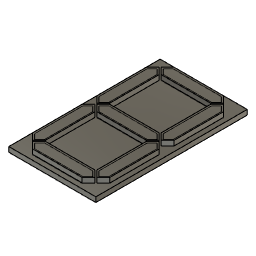
Digit (Autodesk Fusion 360 design; units mm, degrees)
Autodesk Fusion 360 part; units mm, degrees
note: some values were not read from the file. Set by a fixed rule: which face or edge a step refers to.
sketch "Esquisse1" plane through (0, 0, 0) normal (0, 0, 1) x (1, 0, 0)
  line L0 (25, 6.5) -> (-25, 6.5)
  line L1 (-25, 6.5) -> (-25, -6.5)
  line L2 (-25, -6.5) -> (25, -6.5)
  line L3 (25, -6.5) -> (25, 6.5)
  line L4 (25, 6.5) -> (-25, -6.5) construction
  line L5 (-25, 6.5) -> (25, -6.5) construction
  line L6 (-25, 6.5) -> (-25, -6.5) construction
  line L7 (-25, -6.5) -> (-31.5, -6.5) construction
  line L8 (-31.5, -6.5) -> (-31.5, 6.5) construction
  line L9 (-31.5, 6.5) -> (-25, 6.5) construction
  line L10 (-25, 6.5) -> (-31.5, 0)
  line L11 (-25, -6.5) -> (-31.5, 0)
  line L12 (25, 6.5) -> (25, -6.5) construction
  line L13 (25, -6.5) -> (31.5, -6.5) construction
  line L14 (31.5, -6.5) -> (31.5, 6.5) construction
  line L15 (31.5, 6.5) -> (25, 6.5) construction
  line L16 (25, 6.5) -> (31.5, 0)
  line L17 (25, -6.5) -> (31.5, 0)
  line L18 (-25, -6.5) -> (-25, -6.25) construction
  line L19 (-25, -6.25) -> (25, -6.25) construction
  line L20 (25, -6.25) -> (25, -6.5)
  line L21 (25, -6.5) -> (-25, -6.5)
  line L22 (-24.25, -6.25) -> (24.25, -6.25)
  line L23 (24.25, -6.25) -> (24.25, -5)
  line L24 (24.25, -5) -> (-24.25, -5)
  line L25 (-24.25, -5) -> (-24.25, -6.25)
  point P0 (-31.5, 0)
  point P1 (31.5, 0)
  dimension "longueurBande" = 50
  dimension "largeurBande" = 13
  dimension "d3" = 6.5
  dimension "d4" = 6.5
  dimension "d42" = 0.25
  dimension "d50" = 0.75
  dimension "d51" = 48.5
  dimension "d52" = 1.25
  constraint horizontal L0
  constraint perpendicular L0 L1
  constraint parallel L0 L2
  constraint parallel L1 L3
  constraint coincident L4 origin
  constraint coincident L5 origin
  constraint perpendicular L6 L7
  constraint parallel L6 L8
  constraint parallel L7 L9
  constraint midpoint L8 P0
  constraint coincident P0 L10.end
  constraint perpendicular L12 L13
  constraint parallel L12 L14
  constraint parallel L13 L15
  constraint midpoint L14 P1
  constraint coincident P1 L16.end
  constraint perpendicular L18 L19
  constraint parallel L18 L20
  constraint parallel L19 L21
  constraint coincident L1 L18.end
  constraint horizontal L22
  constraint vertical L23
  constraint horizontal L24
  constraint vertical L25
  constraint coincident L19 L22.start
  measures "longueurBande" distance of L1.end L2.end
  measures "largeurBande" distance of L0.end L1.end
  measures "d3" distance of L0.end L8.end
  measures "d4" distance of L0.start L14.end
  measures "d42" distance of L19 L21
  measures "d50" distance of L18.end L22.start
  measures "d51" distance of L23.end L24.end
  measures "d52" distance of L19 L24
extrude "Extrusion1" add sketch "Esquisse1" along normal blind 5 contours L0 L1 L2 L3 L20 L21 | L3 L16 L17 L20 | L1 L10 L11 | L22 L23 L24 L25 makes body 1
shell "Coque2" thickness 1.5 removed faces 1 at (8.3333, 2.1667, 0) on bodies 1
extrude "Extrusion10" cut 1 faces at (-8.1262, -1.6667, 3.5) along direction (0, 0, 1) blind 1 on bodies 1 bodies 1
extrude "Extrusion8" add sketch "Esquisse1" against normal blind 1 contours L22 L23 L24 L25 bodies 1
copy_body "Copier/Coller des corps2" bodies 1 makes body 2
move_body "Déplacer1" bodies 2 to x (0, -1, 0) y (1, 0, 0) z (0, 0, 1) at (-32.5, -32.5, 0)
pattern_linear "Réseau R1" count 3 spacing 65 along (0, -1, 0) of bodies 1 makes body 3 at (-8.3333, -67.1667, 5) makes body 4 at (-8.3333, -132.1667, 5)
pattern_linear "Réseau R2" count 2 spacing 65 along (1, 0, 0) count 2 spacing 65 along (0, -1, 0) of bodies 2 makes body 5 at (34.6667, -40.8333, 5) makes body 6 at (-30.3333, -105.8333, 5) makes body 7 at (34.6667, -105.8333, 5)
sketch "Esquisse2" plane through (0, 0, 0) normal (0, 0, 1) x (1, 0, 0)
  line L0 (-25, -6.5) -> (25, -6.5)
  line L1 (25, -6.5) -> (31.5, 0)
  line L2 (31.5, 0) -> (25, 6.5)
  line L3 (25, 6.5) -> (-25, 6.5)
  line L4 (-25, 6.5) -> (-31.5, 0)
  line L5 (-31.5, 0) -> (-25, -6.5)
  line L6 (26, -7.5) -> (26, -57.5)
  line L7 (26, -57.5) -> (32.5, -64)
  line L8 (32.5, -64) -> (39, -57.5)
  line L9 (39, -57.5) -> (39, -7.5)
  line L10 (39, -7.5) -> (32.5, -1)
  line L11 (32.5, -1) -> (26, -7.5)
  line L12 (-39, -7.5) -> (-39, -57.5)
  line L13 (-39, -57.5) -> (-32.5, -64)
  line L14 (-32.5, -64) -> (-26, -57.5)
  line L15 (-26, -57.5) -> (-26, -7.5)
  line L16 (-26, -7.5) -> (-32.5, -1)
  line L17 (-32.5, -1) -> (-39, -7.5)
  line L18 (-25, -71.5) -> (25, -71.5)
  line L19 (25, -71.5) -> (31.5, -65)
  line L20 (31.5, -65) -> (25, -58.5)
  line L21 (25, -58.5) -> (-25, -58.5)
  line L22 (-25, -58.5) -> (-31.5, -65)
  line L23 (-31.5, -65) -> (-25, -71.5)
  line L24 (-39, -72.5) -> (-39, -122.5)
  line L25 (-39, -122.5) -> (-32.5, -129)
  line L26 (-32.5, -129) -> (-26, -122.5)
  line L27 (-26, -122.5) -> (-26, -72.5)
  line L28 (-26, -72.5) -> (-32.5, -66)
  line L29 (-32.5, -66) -> (-39, -72.5)
  line L30 (26, -72.5) -> (26, -122.5)
  line L31 (26, -122.5) -> (32.5, -129)
  line L32 (32.5, -129) -> (39, -122.5)
  line L33 (39, -122.5) -> (39, -72.5)
  line L34 (39, -72.5) -> (32.5, -66)
  line L35 (32.5, -66) -> (26, -72.5)
  line L36 (-25, -136.5) -> (25, -136.5)
  line L37 (25, -136.5) -> (31.5, -130)
  line L38 (31.5, -130) -> (25, -123.5)
  line L39 (25, -123.5) -> (-25, -123.5)
  line L40 (-25, -123.5) -> (-31.5, -130)
  line L41 (-31.5, -130) -> (-25, -136.5)
  line L42 (-39, 6.5) -> (39, 6.5)
  line L43 (39, 6.5) -> (39, -136.5)
  line L44 (39, -136.5) -> (-39, -136.5)
  line L45 (-39, -136.5) -> (-39, 6.5)
  line L46 (44, 11.5) -> (44, -141.5)
  line L47 (44, -141.5) -> (-44, -141.5)
  line L48 (-44, -141.5) -> (-44, 11.5)
  line L49 (-44, 11.5) -> (44, 11.5)
  line L50 (-25, -6.5) -> (-26, -7.5)
  line L51 (31.5, 0) -> (32.5, -1)
  line L52 (25, -6.5) -> (26, -7.5)
  line L53 (26, -57.5) -> (25, -58.5)
  line L54 (32.5, -64) -> (31.5, -65)
  line L55 (31.5, -65) -> (32.5, -66)
  line L56 (25, -71.5) -> (26, -72.5)
  line L57 (26, -122.5) -> (25, -123.5)
  line L58 (32.5, -129) -> (31.5, -130)
  line L59 (-25, -123.5) -> (-26, -122.5)
  line L60 (-32.5, -129) -> (-31.5, -130)
  line L61 (-32.5, -66) -> (-31.5, -65)
  line L62 (-26, -72.5) -> (-25, -71.5)
  line L63 (-31.5, -65) -> (-32.5, -64)
  line L64 (-25, -58.5) -> (-26, -57.5)
  line L65 (-24.3787, -5) -> (24.3787, -5)
  line L66 (24.3787, -5) -> (29.3787, 0)
  line L67 (29.3787, 0) -> (24.3787, 5)
  line L68 (24.3787, 5) -> (-24.3787, 5)
  line L69 (-24.3787, 5) -> (-29.3787, 0)
  line L70 (-29.3787, 0) -> (-24.3787, -5)
  line L71 (-37.5, -56.8787) -> (-32.5, -61.8787)
  line L72 (-32.5, -61.8787) -> (-27.5, -56.8787)
  line L73 (-27.5, -56.8787) -> (-27.5, -8.1213)
  line L74 (-27.5, -8.1213) -> (-32.5, -3.1213)
  line L75 (-32.5, -3.1213) -> (-37.5, -8.1213)
  line L76 (-37.5, -8.1213) -> (-37.5, -56.8787)
  line L77 (27.5, -56.8787) -> (32.5, -61.8787)
  line L78 (32.5, -61.8787) -> (37.5, -56.8787)
  line L79 (37.5, -56.8787) -> (37.5, -8.1213)
  line L80 (37.5, -8.1213) -> (32.5, -3.1213)
  line L81 (32.5, -3.1213) -> (27.5, -8.1213)
  line L82 (27.5, -8.1213) -> (27.5, -56.8787)
  line L83 (-24.3787, -70) -> (24.3787, -70)
  line L84 (24.3787, -70) -> (29.3787, -65)
  line L85 (29.3787, -65) -> (24.3787, -60)
  line L86 (24.3787, -60) -> (-24.3787, -60)
  line L87 (-24.3787, -60) -> (-29.3787, -65)
  line L88 (-29.3787, -65) -> (-24.3787, -70)
  line L89 (27.5, -121.8787) -> (32.5, -126.8787)
  line L90 (32.5, -126.8787) -> (37.5, -121.8787)
  line L91 (37.5, -121.8787) -> (37.5, -73.1213)
  line L92 (37.5, -73.1213) -> (32.5, -68.1213)
  line L93 (32.5, -68.1213) -> (27.5, -73.1213)
  line L94 (27.5, -73.1213) -> (27.5, -121.8787)
  line L95 (-37.5, -121.8787) -> (-32.5, -126.8787)
  line L96 (-32.5, -126.8787) -> (-27.5, -121.8787)
  line L97 (-27.5, -121.8787) -> (-27.5, -73.1213)
  line L98 (-27.5, -73.1213) -> (-32.5, -68.1213)
  line L99 (-32.5, -68.1213) -> (-37.5, -73.1213)
  line L100 (-37.5, -73.1213) -> (-37.5, -121.8787)
  line L101 (-24.3787, -135) -> (24.3787, -135)
  line L102 (24.3787, -135) -> (29.3787, -130)
  line L103 (29.3787, -130) -> (24.3787, -125)
  line L104 (24.3787, -125) -> (-24.3787, -125)
  line L105 (-24.3787, -125) -> (-29.3787, -130)
  line L106 (-29.3787, -130) -> (-24.3787, -135)
  line L107 (-32.5, -3.1213) -> (-29.3787, 0)
  line L108 (-24.3787, -5) -> (-27.5, -8.1213)
  line L109 (24.3787, -5) -> (27.5, -8.1213)
  line L110 (32.5, -3.1213) -> (29.3787, 0)
  line L111 (27.5, -56.8787) -> (24.3787, -60)
  line L112 (32.5, -61.8787) -> (32.5, -68.1213)
  line L113 (27.5, -73.1213) -> (24.3787, -70)
  line L114 (27.5, -121.8787) -> (24.3787, -125)
  line L115 (32.5, -126.8787) -> (29.3787, -130)
  line L116 (-27.5, -121.8787) -> (-24.3787, -125)
  line L117 (-29.3787, -130) -> (-32.5, -126.8787)
  line L118 (-32.5, -61.8787) -> (-32.5, -68.1213)
  line L119 (-27.5, -73.1213) -> (-24.3787, -70)
  line L120 (-24.3787, -60) -> (-27.5, -56.8787)
  line L121 (-32.5, -68.1213) -> (-32.5, -61.8787)
  line L122 (-32.5, -61.8787) -> (-39, -61.8787)
  line L123 (-39, -61.8787) -> (-39, -68.1213)
  line L124 (-39, -68.1213) -> (-32.5, -68.1213)
  line L125 (32.5, -68.1213) -> (32.5, -61.8787)
  line L126 (32.5, -61.8787) -> (39, -61.8787)
  line L127 (39, -61.8787) -> (39, -68.1213)
  line L128 (39, -68.1213) -> (32.5, -68.1213)
  line L129 (-24.3787, 5) -> (24.3787, 5)
  line L130 (24.3787, 5) -> (24.3787, 6.5)
  line L131 (24.3787, 6.5) -> (-24.3787, 6.5)
  line L132 (-24.3787, 6.5) -> (-24.3787, 5)
  line L133 (-37.5, -8.1213) -> (-37.5, -56.8787)
  line L134 (-37.5, -56.8787) -> (-39, -56.8787)
  line L135 (-39, -56.8787) -> (-39, -8.1213)
  line L136 (-39, -8.1213) -> (-37.5, -8.1213)
  line L137 (-24.3787, -135) -> (24.3787, -135)
  line L138 (24.3787, -135) -> (24.3787, -136.5)
  line L139 (24.3787, -136.5) -> (-24.3787, -136.5)
  line L140 (-24.3787, -136.5) -> (-24.3787, -135)
  line L141 (37.5, -121.8787) -> (37.5, -73.1213)
  line L142 (37.5, -73.1213) -> (39, -73.1213)
  line L143 (39, -73.1213) -> (39, -121.8787)
  line L144 (39, -121.8787) -> (37.5, -121.8787)
  line L145 (37.5, -56.8787) -> (37.5, -8.1213)
  line L146 (37.5, -8.1213) -> (39, -8.1213)
  line L147 (39, -8.1213) -> (39, -56.8787)
  line L148 (39, -56.8787) -> (37.5, -56.8787)
  line L149 (-37.5, -121.8787) -> (-37.5, -73.1213)
  line L150 (-37.5, -73.1213) -> (-39, -73.1213)
  line L151 (-39, -73.1213) -> (-39, -121.8787)
  line L152 (-39, -121.8787) -> (-37.5, -121.8787)
  line L153 (-24.3787, -70) -> (24.3787, -70)
  line L154 (24.3787, -70) -> (24.3787, -71.5)
  line L155 (24.3787, -71.5) -> (-24.3787, -71.5)
  line L156 (-24.3787, -71.5) -> (-24.3787, -70)
  dimension "d18" = 78
  dimension "d19" = 143
  dimension "d20" = -5
  dimension "d22" = -1.5
  dimension "d23" = -1.5
  dimension "d24" = -1.5
  dimension "d25" = -1.5
  dimension "d26" = -1.5
  dimension "d27" = -1.5
  dimension "d28" = -1.5
  constraint horizontal L42
  constraint vertical L43
  constraint horizontal L44
  constraint vertical L45
  constraint collinear L3 L42
  constraint collinear L12 L45
  constraint coincident L0.start L5.end
  constraint coincident L15.end L16.start
  constraint coincident L1.end L2.start
  constraint coincident L10.end L11.start
  constraint coincident L0.end L1.start
  constraint coincident L6.start L11.end
  constraint coincident L6.end L7.start
  constraint coincident L20.end L21.start
  constraint coincident L7.end L8.start
  constraint coincident L19.end L20.start
  constraint coincident L34.end L35.start
  constraint coincident L18.end L19.start
  constraint coincident L30.start L35.end
  constraint coincident L30.end L31.start
  constraint coincident L38.end L39.start
  constraint coincident L31.end L32.start
  constraint coincident L37.end L38.start
  constraint coincident L39.end L40.start
  constraint coincident L26.end L27.start
  constraint coincident L25.end L26.start
  constraint coincident L40.end L41.start
  constraint coincident L28.end L29.start
  constraint coincident L22.end L23.start
  constraint coincident L27.end L28.start
  constraint coincident L18.start L23.end
  constraint coincident L13.end L14.start
  constraint coincident L21.end L22.start
  constraint coincident L14.end L15.start
  constraint perpendicular L121 L122
  constraint parallel L121 L123
  constraint parallel L122 L124
  constraint perpendicular L125 L126
  constraint parallel L125 L127
  constraint parallel L126 L128
  constraint perpendicular L129 L130
  constraint parallel L129 L131
  constraint parallel L130 L132
  constraint perpendicular L133 L134
  constraint parallel L133 L135
  constraint parallel L134 L136
  constraint perpendicular L137 L138
  constraint parallel L137 L139
  constraint parallel L138 L140
  constraint perpendicular L141 L142
  constraint parallel L141 L143
  constraint parallel L142 L144
  constraint perpendicular L145 L146
  constraint parallel L145 L147
  constraint parallel L146 L148
  constraint perpendicular L149 L150
  constraint parallel L149 L151
  constraint parallel L150 L152
  constraint perpendicular L153 L154
  constraint parallel L153 L155
  constraint parallel L154 L156
  measures "d18" distance of L42.start L42.end
  measures "d19" distance of L42.start L44.end
extrude "Extrusion2" add sketch "Esquisse2" against normal blind 5 separate body contours L0 L1 L5 L65 L108 L109 | L5 L16 L50 L108 | L0 L6 L15 L21 L50 L52 L53 L64 | L1 L11 L52 L109 | L14 L15 L16 L73 L108 L120 | L6 L7 L11 L82 L109 L111 | L14 L22 L64 L120 | L7 L20 L53 L111 | L20 L21 L22 L86 L111 L120 | L3 L42 L68 L129 L130 L131 L132 | L12 L45 L76 L133 L134 L135 L136 | L9 L43 L79 L145 L146 L147 L148 | L18 L23 L119 L156 | L23 L28 L62 L119 | L26 L27 L28 L97 L116 L119 | L19 L35 L56 L113 | L18 L19 L113 L154 | L30 L31 L35 L94 L113 L114 | L18 L27 L30 L39 L56 L57 L59 L62 L155 | L18 L83 L153 L154 L155 L156 | L24 L45 L100 L149 L150 L151 L152 | L33 L43 L91 L141 L142 L143 L144 | L26 L40 L59 L116 | L31 L38 L57 L114 | L38 L39 L40 L104 L114 L116 | L36 L44 L101 L137 L138 L139 L140 | L46 L47 L48 L49 makes body 8 at (-9.1667, -89.3738, 0) makes body 9 at (8.1262, -23.3333, 0) makes body 10 at (42.3333, -62.2929, 0)
extrude "Extrusion4" add sketch "Esquisse2" against normal blind 2.5 contours L5 L16 L107 L108 | L5 L70 L107 L108 | L1 L66 L109 L110 | L1 L11 L109 L110 | L4 L5 L16 L17 L42 L45 L107 | L3 L4 L5 L42 L69 L107 L132 | L16 L74 L107 L108 | L1 L2 L3 L42 L67 L110 L130 | L1 L11 L51 L110 | L11 L81 L109 L110 | L12 L16 L17 L45 L75 L107 L136 | L14 L22 L63 L120 | L14 L72 L118 L120 L121 | L2 L10 L42 L43 L51 | L9 L10 L11 L43 L80 L110 L146 | L7 L77 L111 L112 L125 | L7 L20 L54 L111 | L13 L29 L45 L118 L121 L122 L123 L124 | L13 L118 L121 L122 | L61 L63 L118 L121 | L22 L23 L87 L88 L119 L120 | L8 L112 L125 L126 | L54 L55 L112 L125 | L8 L34 L43 L112 L125 L126 L127 L128 | L19 L20 L84 L85 L111 L113 | L12 L13 L45 L71 L122 L134 | L13 L45 L122 | L23 L28 L61 L119 | L29 L118 L121 L124 | L28 L98 L118 L119 L121 | L8 L9 L43 L78 L126 L148 | L8 L43 L126 | L19 L35 L55 L113 | L35 L93 L112 L113 L125 | L34 L112 L125 L128 | L24 L29 L45 L99 L124 L150 | L29 L45 L124 | L34 L43 L128 | L33 L34 L43 L92 L128 L142 | L26 L96 L116 L117 | L24 L25 L26 L45 L95 L117 L152 | L31 L89 L114 L115 | L31 L32 L33 L43 L90 L115 L144 | L26 L40 L116 L117 | L31 L38 L114 L115 | L26 L40 L60 L117 | L40 L105 L116 L117 | L25 L41 L44 L45 L60 | L32 L37 L43 L44 L58 | L31 L38 L58 L115 | L38 L103 L114 L115 | L36 L40 L41 L44 L106 L117 L140 | L36 L37 L38 L44 L102 L115 L138 bodies 8 10 9
extrude "Extrusion9" cut sketch "Esquisse2" against normal blind 1 contours L3 L42 L68 L129 L130 L131 L132 | L12 L45 L76 L133 L134 L135 L136 | L9 L43 L79 L145 L146 L147 L148 | L18 L83 L153 L154 L155 L156 | L24 L45 L100 L149 L150 L151 L152 | L33 L43 L91 L141 L142 L143 L144 | L36 L44 L101 L137 L138 L139 L140 bodies 8
equation "largeurBande = 10 mm + margeDigit"
equation "d3 = largeurBande / 2"
equation "d4 = largeurBande / 2"
equation "d9 = -longueurBande - largeurBande - espacement * 2"
equation "d13 = largeurBande + longueurBande + espacement * 2"
equation "d14 = -largeurBande - longueurBande - espacement * 2"
equation "espacement = 1 mm"
equation "d18 = longueurBande + largeurBande * 2 + espacement * 2"
equation "d19 = longueurBande * 2 + largeurBande * 3 + espacement * 4"
equation "margeDigit = 3 mm"
equation "d22 = -margeDigit / 2"
equation "d23 = -margeDigit / 2"
equation "d24 = -margeDigit / 2"
equation "d25 = -margeDigit / 2"
equation "d26 = -margeDigit / 2"
equation "d27 = -margeDigit / 2"
equation "d28 = -margeDigit / 2"
equation "d45 = margeDigit / 2"
equation "d51 = longueurBande - 1.5 mm"
equation "d52 = 1.5 mm - 0.25 mm"
named bodies: "Base"
